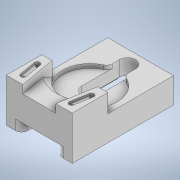
# Autodesk Inventor part: Część15
Saved by Autodesk Inventor 2021 (Build 250183000, 183)
## iProperties
Created: 2023-10-18
Part Number: Część15
Material: Ogólny
Document SubType Name: Modeling
Designer: Jakub
Density: 1 g/cm^3
Appearance: Domyślna
Author: Jakub
Autodesk Inventor part; units mm, degrees
ref_plane "YZ Plane" through (0, 0, 0) normal (1, 0, 0) x (0, 1, 0)
ref_plane "XZ Plane" through (0, 0, 0) normal (0, 1, 0) x (-1, 0, 0)
ref_plane "XY Plane" through (0, 0, 0) normal (0, 0, 1) x (1, 0, 0)
sketch "Szkic1" plane through (0, 0, 0) normal (0, 1, 0) x (-1, 0, 0)
  line L0 (0, 0) -> (0, -100)
  line L1 (0, -100) -> (-65, -100)
  line L2 (-65, -100) -> (-65, 0)
  line L3 (-65, 0) -> (0, 0)
  dimension "d0" = 100
  dimension "d1" = 65
  constraints: 8 end point, 3 perpendicular, 1 vertical
  measures "d0" distance of L0.start L0.end
  measures "d1" distance of L0.end L1.end
extrude "Wyciągnięcie proste1" add sketch "Szkic1" along normal blind 15
sketch "Szkic3" plane through (0, 0, 0) normal (0, -1, 0) x (1, 0, 0)
  line L0 (0, 0) -> (65, 0) projected
  line L1 (32.5, 0) -> (32.5, -100)
  line L2 (65, -100) -> (0, -100) projected
  line L3 (32.5, -50) -> (15, -50)
  line L4 (15, -50) -> (50, -50)
  line L5 (50, -50) -> (50, 0)
  line L6 (65, 0) -> (65, -100) projected
  line L7 (50, 0) -> (65, 0)
  line L8 (65, 0) -> (65, -100)
  line L9 (65, -100) -> (50, -100)
  line L10 (50, -100) -> (50, -50)
  line L11 (15, -50) -> (15, -100)
  line L12 (15, -100) -> (0, -100)
  line L13 (0, -100) -> (0, 0) projected
  line L14 (0, -100) -> (0, 0)
  line L15 (0, 0) -> (15, 0)
  line L16 (15, -50) -> (15, 0)
  dimension "d4" = 17.5
  dimension "d5" = 35
  constraints: 26 end point, 6 point on line, 5 perpendicular, 3 midpoint, 2 parallel, 1 collinear, 1 horizontal
  measures "d4" distance of L3.start L3.end
  measures "d5" distance of L3.end L4.end
extrude "Wyciągnięcie proste2" add sketch "Szkic3" along normal blind 10 contours L0 L16 L11 L2 L13 | L0 L6 L2 L10 L5
fillet "Zaokrąglenie1" radius 6 4 edges at (15, -5, -100) (15, -5, 0) (50, -5, 0) (50, -5, -100)
sketch "Szkic4" plane through (0, 15, 0) normal (0, 1, 0) x (1, 0, 0)
  line L0 (0, 0) -> (0, 35)
  line L1 (0, 0) -> (0, 100) projected
  line L2 (0, 35) -> (65, 35)
  line L3 (65, 100) -> (65, 0) projected
  line L4 (0, 0) -> (65, 0) projected
  line L5 (65, 0) -> (65, 35)
  line L6 (0, 0) -> (65, 0)
  line L7 (9, 0) -> (56, 0) projected
  dimension "d9" = 35
  constraints: 8 end point, 2 perpendicular, 2 point on line, 1 collinear
  measures "d9" distance of L0.start L0.end
extrude "Wyciągnięcie proste3" add sketch "Szkic4" along normal blind 10
sketch "Szkic5" plane through (0, 25, 0) normal (0, 1, 0) x (1, 0, 0)
  line L0 (0, 0) -> (32.5, 0)
  line L1 (9, 0) -> (56, 0) projected
  line L2 (32.5, 0) -> (32.5, 100)
  line L3 (56, 100) -> (9, 100) projected
  line L4 (0, 35) -> (65, 35) projected
  line L5 (32.5, 35) -> (10, 35)
  line L6 (10, 35) -> (55, 35)
  line L7 (55, 35) -> (55, 0)
  line L8 (10, 35) -> (10, 0)
  line L9 (10, 35) -> (16.1714, 0)
  line L10 (10, 35) -> (45.5399, 35) construction
  line L11 (55, 35) -> (48.8286, 0)
  line L12 (55, 35) -> (90.5399, 35) construction
  line L13 (65, 0) -> (65, 35) projected
  line L14 (55, 0) -> (65, 0)
  line L15 (65, 0) -> (65, 35)
  line L16 (55, 35) -> (65, 35)
  line L17 (10, 35) -> (0, 35)
  line L18 (0, 35) -> (0, 0) projected
  line L19 (0, 0) -> (10, 0)
  line L20 (9, 0) -> (0, 0) projected
  line L21 (0, 0) -> (0, 35)
  line L22 (0, 0) -> (0, 100) projected
  dimension "d12" = 22.5
  dimension "d13" = 45
  dimension "d14" = 80
  dimension "d15" = 100
  constraints: 32 end point, 6 point on line, 4 collinear, 3 midpoint, 3 perpendicular, 2 equal length, 2 horizontal, 1 vertical
  measures "d12" distance of L5.start L5.end
  measures "d13" distance of L5.end L6.end
  measures "d14" angle of L9 L10
  measures "d15" angle of L11 L12
extrude "Wyciągnięcie proste4" add sketch "Szkic5" along normal blind 8 contours L18 L4 L8 L0 | L8 L9 L0 | L4 L13 L14 L1 L7 | L7 L1 L11
sketch "Szkic6" plane through (0, 15, 0) normal (0, 1, 0) x (1, 0, 0)
  line L0 (56, 100) -> (9, 100) projected
  line L1 (32.5, 100) -> (32.5, 0)
  line L2 (32.5, 0) -> (32.5, 50)
  line L3 (32.5, 50) -> (0, 50)
  line L4 (0, 0) -> (0, 100) projected
  line L5 (32.5, 50) -> (65, 50)
  line L6 (65, 35) -> (65, 100) projected
  circle A0 centre (32.5, 50) radius 27.0416
  point P0 (10, 35)
  constraints: 8 end point, 3 midpoint, 2 point on line, 1 coincident, 1 vertical, 3 other
extrude "Wyciągnięcie proste5" cut sketch "Szkic6" along normal blind 15 and the other way blind 4
chamfer "Faza1" distance 6 angle 45 1 edges at (32.5, 25, -22.9584)
sketch "Szkic7" plane through (0, 0, 0) normal (0, -1, 0) x (1, 0, 0)
  line L0 (16.1714, 0) -> (48.8286, 0) projected
  line L1 (32.5, 0) -> (32.5, -100)
  line L2 (65, -100) -> (0, -100) projected
  line L3 (32.5, -50) -> (0, -50)
  line L4 (0, -50) -> (0, -87)
  line L5 (0, -100) -> (0, -35) projected
  line L6 (0, -87) -> (32.5, -87)
  circle A0 centre (32.5, -50) radius 8
  circle A1 centre (32.5, -87) radius 8
  line L7 (40.5, -50) -> (40.5, -87)
  line L8 (24.5, -87) -> (24.5, -50)
  point P0 (0, 0)
  dimension "d25" = 37
  dimension "d26" = 16
  dimension "d27" = 16
  constraints: 12 end point, 4 point on circle, 4 point on line, 3 midpoint, 2 centre point, 2 coincident, 1 horizontal, 1 perpendicular, 1 tangent
  measures "d25" distance of L3.end L4.end
  measures "d26" diameter of A0
  measures "d27" diameter of A1
extrude "Wyciągnięcie proste6" cut sketch "Szkic7" against normal blind 15 contours A0 L1 | L1 L3 A0 | L1 A0 L3 | L7 A1 L1 A0 | A0 L1 A1 L8 | A1 L1 | A1 L1 L6 | L6 L1 A1
fillet "Zaokrąglenie2" radius 6 2 edges at (24.5, 13, -75.8312) (40.5, 13, -75.8312)
sketch "Szkic8" plane through (0, 33, 0) normal (0, 1, 0) x (1, 0, 0)
  line L0 (55, 35) -> (48.8286, 0) projected
  line L1 (51.9929, 17.9457) -> (57.9017, 16.9038)
  line L2 (51.9929, 17.9457) -> (57.9929, 17.9457) construction
  line L3 (57.9017, 16.9038) -> (61.0926, 35)
  line L4 (65, 35) -> (55, 35) projected
  line L5 (57.9017, 16.9038) -> (54.9211, 0)
  line L6 (65, 0) -> (56, 0) projected
  line L7 (48.8286, 0) -> (65, 0) projected
  line L8 (50.9367, 0) -> (50.9367, 8)
  line L9 (50.9367, 0) -> (58.9367, 0) construction
  line L10 (50.9367, 8) -> (65, 8)
  line L11 (65, 0) -> (65, 35) projected
  circle A0 centre (56.3317, 8) radius 2.5
  line L12 (56.3317, 8) -> (59.2838, 24.7417)
  circle A1 centre (59.2838, 24.7417) radius 2.5
  line L13 (53.8317, 8) -> (56.8208, 25.1705)
  line L14 (58.8317, 8) -> (61.7448, 24.302)
  point P0 (0, 0)
  dimension "d31" = 6
  dimension "d32" = 10
  dimension "d33" = 8
  dimension "d34" = 90
  dimension "d35" = 5
  dimension "d36" = 17
  dimension "d37" = 5
  constraints: 20 end point, 11 point on line, 4 perpendicular, 4 point on circle, 2 centre point, 2 equal length, 2 horizontal, 2 tangent, 1 coincident
  measures "d31" distance of L1.start L1.end
  measures "d32" angle of L1 L2
  measures "d33" distance of L8.start L8.end
  measures "d34" angle of L9 L8
  measures "d35" diameter of A0
  measures "d36" distance of L12.start L12.end
  measures "d37" diameter of A1
extrude "Wyciągnięcie proste7" cut sketch "Szkic8" against normal blind 2 contours L13 A1 L3 L1 | L1 L5 A0 L13 | A1 L3 | L3 A1 | L3 A1 L14 A0 L5 | A0 L5 L10 L13 | A0 L10 L5 | L10 L5 A0 | A0 L5 L10
sketch "Szkic9" plane through (0, 33, 0) normal (0, 1, 0) x (1, 0, 0)
  line L0 (16.1714, 0) -> (10, 35) projected
  line L1 (12.5503, 20.5363) -> (6.6415, 19.4944)
  line L2 (12.5503, 20.5363) -> (18.5503, 20.5363) construction
  line L3 (6.6415, 19.4944) -> (3.9074, 35)
  line L4 (0, 35) -> (10, 35) projected
  line L5 (6.6415, 19.4944) -> (10.0622, 0.0948)
  line L6 (10.0622, 0.0948) -> (10.0622, 8.0948)
  line L7 (0, 35) -> (0, 0) projected
  line L8 (8.6516, 8.0948) -> (5.6995, 24.8365)
  circle A0 centre (8.6516, 8.0948) radius 2.5
  circle A1 centre (5.6995, 24.8365) radius 2.5
  line L9 (8.1616, 25.2706) -> (11.1136, 8.5289)
  line L10 (6.1895, 7.6606) -> (3.2375, 24.4024)
  dimension "d40" = 6
  dimension "d41" = 170
  dimension "d42" = 8
  dimension "d43" = 17
  dimension "d44" = 5
  dimension "d45" = 5
  constraints: 16 end point, 5 point on line, 4 point on circle, 3 tangent, 2 centre point, 2 coincident, 2 perpendicular, 1 equal length, 1 horizontal, 1 vertical
  measures "d40" distance of L1.start L1.end
  measures "d41" angle of L1 L2
  measures "d42" distance of L5.end L6.end
  measures "d43" distance of L8.start L8.end
  measures "d44" diameter of A0
  measures "d45" diameter of A1
extrude "Wyciągnięcie proste8" cut sketch "Szkic9" against normal blind 2 contours L9 A0 L5 L1 | L1 L3 A1 L9 | L5 A0 L10 A1 L3 | A1 L3 | A0 L5 | L3 A1 | L5 A0
sketch "Szkic10" plane through (0, 31, 0) normal (0, 1, 0) x (1, 0, 0)
  arc A0 (8.1616, 25.2706) -> (3.2375, 24.4024) centre (5.6995, 24.8365) ccw projected
  arc A1 (6.1895, 7.6606) -> (11.1136, 8.5289) centre (8.6516, 8.0948) ccw projected
  line L0 (5.6995, 24.8365) -> (8.6516, 8.0948)
  circle A2 centre (8.6516, 8.0948) radius 1.5
  circle A3 centre (5.6995, 24.8365) radius 1.5
  arc A4 (53.8317, 8) -> (58.8317, 8) centre (56.3317, 8) ccw projected
  arc A5 (61.7448, 24.302) -> (56.8208, 25.1705) centre (59.2838, 24.7417) ccw projected
  line L1 (56.3317, 8) -> (59.2838, 24.7417)
  circle A6 centre (56.3317, 8) radius 1.5
  circle A7 centre (59.2838, 24.7417) radius 1.5
  point P0 (0, 0)
  dimension "d48" = 3
  dimension "d49" = 3
  dimension "d50" = 3
  dimension "d51" = 3
  constraints: 4 centre point, 4 coincident, 4 end point
  measures "d48" diameter of A2
  measures "d49" diameter of A3
  measures "d50" diameter of A6
  measures "d51" diameter of A7
extrude "Wyciągnięcie proste9" cut sketch "Szkic10" against normal blind 41
